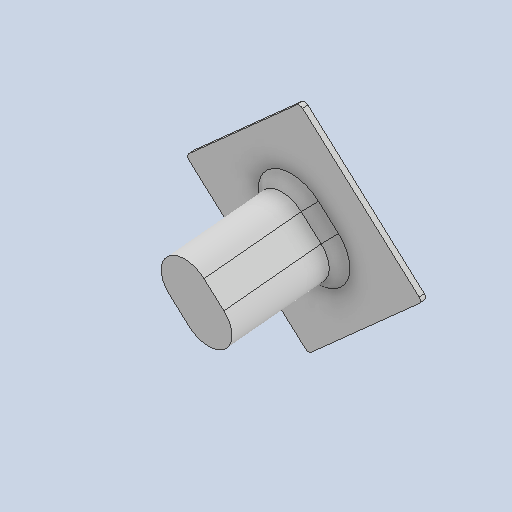
# Autodesk Inventor part: Staging_area
Saved by Autodesk Inventor 2024 (Build 280153000, 153)
## iProperties
Created: 2023-06-25
Part Number: Staging_area
Material: Generic
Document SubType Name: Modeling
Designer: Rober
Density: 1 g/cm^3
Appearance: Default
Author: Rober
Autodesk Inventor part; units mm, degrees
ref_plane "YZ Plane" through (0, 0, 0) normal (1, 0, 0) x (0, 1, 0)
ref_plane "XZ Plane" through (0, 0, 0) normal (0, 1, 0) x (-1, 0, 0)
ref_plane "Work Plane1" through (-49.3077, -59.6436, 136.7512) normal (-0.0070087, 0.0889934, -0.9960076) x (-0.7423447, -0.6678024, -0.0544445)
sketch "Sketch1" plane through (-49.3077, -59.6436, 136.7512) normal (-0.0070087, 0.0889934, -0.9960076) x (-0.7423447, -0.6678024, -0.0544445)
  arc A0 (12.185, 6.495) -> (-12.185, 6.495) centre (0, 6.495) ccw projected
  arc A1 (12.185, 6.495) -> (-12.185, 6.495) centre (0, 6.495) ccw projected
  line L0 (-12.185, -6.495) -> (-12.185, 6.495) projected
  arc A2 (-12.185, -6.495) -> (12.185, -6.495) centre (0, -6.495) ccw projected
  arc A3 (-12.185, -6.495) -> (12.185, -6.495) centre (0, -6.495) ccw projected
  line L1 (12.185, 6.495) -> (12.185, -6.495) projected
  line L2 (-10.685, -6.495) -> (-10.685, 6.005)
  arc A4 (10.685, 6.495) -> (-10.685, 6.495) centre (0, 6.495) ccw
  arc A5 (-10.685, -6.495) -> (10.685, -6.495) centre (0, -6.495) ccw
  line L3 (10.685, 6.495) -> (10.685, -6.005)
  point P0 (-68.9881, 1.367)
  point P1 (10.685, 6.495)
  point P2 (10.5, -6.25)
  point P3 (-10.685, -6.495)
  point P4 (-10.5, 6.25)
  dimension "d0" = 1.5
  dimension "d1" = 1.5
  dimension "d2" = 1.5
  dimension "d3" = 1.5
  constraints: 4 end point, 4 point on circle, 2 centre point, 2 parallel
  measures "d0" distance between parallel lines of L0 L2
  measures "d1" radial gap between concentric circles of A0 A4
  measures "d2" radial gap between concentric circles of A2 A5
  measures "d3" distance between parallel lines of L1 L3
extrude "Extrusion1" add sketch "Sketch1" along normal blind 50
sketch "Sketch2" plane through (-49.6582, -55.1939, 86.9509) normal (-0.0070087, 0.0889934, -0.9960076) x (-0.7423447, -0.6678024, -0.0544445)
  arc A0 (12.185, 6.495) -> (-12.185, 6.495) centre (0, 6.495) ccw projected
  line L0 (12.185, -6.495) -> (12.185, 6.495) projected
  arc A1 (-12.185, -6.495) -> (12.185, -6.495) centre (0, -6.495) ccw projected
  line L1 (-12.185, 6.495) -> (-12.185, -6.495) projected
  point P0 (-68.9881, 1.367)
extrude "Extrusion2" add sketch "Sketch2" along normal blind 2.5
sketch "Sketch3" plane through (-49.6757, -54.9714, 84.4608) normal (-0.0070087, 0.0889934, -0.9960076) x (-0.7423447, -0.6678024, -0.0544445)
  line L0 (-38, 40) -> (38, 40)
  line L1 (40, 38) -> (40, -38)
  line L2 (38, -40) -> (-38, -40)
  line L3 (-40, -38) -> (-40, 38)
  arc A0 (12.185, 6.495) -> (-12.185, 6.495) centre (0, 6.495) ccw projected
  line L4 (0, 40) -> (0, 18.68)
  arc A1 (-12.185, -6.495) -> (12.185, -6.495) centre (0, -6.495) ccw projected
  line L5 (0, -18.68) -> (0, -40)
  line L6 (-12.185, 6.495) -> (-12.185, -6.495) projected
  line L7 (-12.185, 0) -> (-40, 0)
  line L8 (12.185, -6.495) -> (12.185, 6.495) projected
  line L9 (12.185, 0) -> (40, 0)
  arc A2 (-38, 40) -> (-40, 38) centre (-38, 38) ccw
  arc A3 (40, 38) -> (38, 40) centre (38, 38) ccw
  arc A4 (-40, -38) -> (-38, -40) centre (-38, -38) ccw
  arc A5 (38, -40) -> (40, -38) centre (38, -38) ccw
  point P0 (-68.9881, 1.367)
  point P1 (-40, 40)
  point P2 (40, -40)
  point P3 (-40, -40)
  dimension "d8" = 80
  dimension "d9" = 80
  dimension "d11" = 2
  dimension "d12" = 2
  dimension "d13" = 2
  dimension "d14" = 2
  constraints: 16 end point, 10 point on circle, 8 point on line, 8 tangent, 6 midpoint, 4 centre point, 2 parallel, 2 perpendicular, 1 collinear, 1 horizontal, 1 vertical
  measures "d8" distance of point (-40, -40) point (-40, 40)
  measures "d9" distance of point (40, -40) point (-40, -40)
  measures "d11" radius of A2
  measures "d12" radius of A3
  measures "d13" radius of A4
  measures "d14" radius of A5
extrude "Extrusion3" add sketch "Sketch3" along normal blind 2.5
chamfer "Chamfer1" distance 5 angle 45 4 edges at (-58.7212, -63.1086, 83.7974) (-62.1909, -41.1669, 85.7823) (-40.6302, -46.8343, 85.1242) (-37.1604, -68.7759, 83.1393)
body "Solid1"
